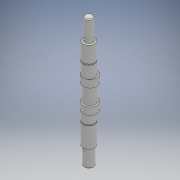
# Autodesk Inventor part: 도면2-4번
Saved by Autodesk Inventor 2018.3 (Build 223284000, 284)
## iProperties
Created: 2019-10-11
Part Number: 도면2-4번
Material: 일반
Document SubType Name: Modeling
Designer: MyTool
Density: 1 g/cm^3
Appearance: 기본값
Author: MyTool
Autodesk Inventor part; units mm, degrees
ref_plane "YZ Plane" through (0, 0, 0) normal (1, 0, 0) x (0, 1, 0)
ref_plane "XZ Plane" through (0, 0, 0) normal (0, 1, 0) x (-1, 0, 0)
ref_plane "XY Plane" through (0, 0, 0) normal (0, 0, 1) x (1, 0, 0)
sketch "스케치1" plane through (0, 0, 0) normal (1, 0, 0) x (0, 1, 0)
  line L0 (0, 0) -> (6, 0)
  line L1 (6, 0) -> (6, 23)
  line L2 (6, 23) -> (0, 23)
  line L3 (0, 23) -> (0, 0)
  line L4 (0, 23) -> (7.5, 23)
  line L5 (7.5, 23) -> (7.5, 61)
  line L6 (7.5, 61) -> (0, 61)
  line L7 (0, 61) -> (0, 23)
  line L8 (0, 61) -> (10.5, 61)
  line L9 (10.5, 61) -> (10.5, 70.5)
  line L10 (10.5, 70.5) -> (0, 70.5)
  line L11 (0, 70.5) -> (0, 61)
  line L12 (0, 70.5) -> (12.5, 70.5)
  line L13 (12.5, 70.5) -> (12.5, 91.5)
  line L14 (12.5, 91.5) -> (0, 91.5)
  line L15 (0, 91.5) -> (0, 70.5)
  line L16 (0, 91.5) -> (10.5, 91.5)
  line L17 (10.5, 91.5) -> (10.5, 101)
  line L18 (10.5, 101) -> (0, 101)
  line L19 (0, 101) -> (0, 91.5)
  line L20 (0, 101) -> (7.5, 101)
  line L21 (7.5, 101) -> (7.5, 139)
  line L22 (7.5, 139) -> (0, 139)
  line L23 (0, 139) -> (0, 101)
  line L24 (0, 139) -> (5, 139)
  line L25 (5, 139) -> (5, 166)
  line L26 (5, 166) -> (0, 166)
  line L27 (0, 166) -> (0, 139)
  dimension "d0" = 23
  dimension "d1" = 38
  dimension "d2" = 9.5
  dimension "d3" = 21
  dimension "d4" = 9.5
  dimension "d5" = 38
  dimension "d6" = 27
  dimension "d7" = 12
  dimension "d8" = 15
  dimension "d9" = 21
  dimension "d10" = 25
  dimension "d11" = 10
  constraints: 56 end point, 14 parallel, 7 horizontal, 7 perpendicular, 2 point on line
  measures "d0" distance of L0.end L1.end
  measures "d1" distance of L4.end L5.end
  measures "d2" distance of L8.end L9.end
  measures "d3" distance of L12.end L13.end
  measures "d4" distance of L16.end L17.end
  measures "d5" distance of L20.end L21.end
  measures "d6" distance of L24.end L25.end
  measures "d7" diameter of L1 L3
  measures "d8" diameter of L5 L7
  measures "d9" diameter of L9 L11
  measures "d10" diameter of L13 L15
  measures "d11" diameter of L25 L27
revolve "회전1" add sketch "스케치1" angle 360 about axis through (0, 0, 23) along (0, 0, -1)
sketch "스케치3" plane through (0, 0, 101) normal (0, 0, 1) x (1, 0, 0)
  circle A0 centre (0, 0) radius 7.5 projected
  circle A1 centre (0, 1.5) radius 9
  circle A2 centre (0, 0) radius 10.5 projected
  dimension "d13" = 18
  constraints: 1 centre point, 1 tangent
  measures "d13" diameter of A1
extrude "돌출1" cut sketch "스케치3" against normal blind 9.5 contours A2
sketch "스케치2" plane through (0, 0, 61) normal (0, 0, -1) x (-1, 0, 0)
  circle A0 centre (0, 1.5) radius 9 projected
  circle A1 centre (0, 0) radius 10.5 projected
  point P0 (0, -7.5)
  constraints: 1 vertical alignment
extrude "돌출2" cut sketch "스케치2" against normal blind 9.5
sketch "스케치4" plane through (0, 0, 70.5) normal (0, 0, -1) x (-1, 0, 0)
  circle A0 centre (0, 1.5) radius 9 projected
  circle A1 centre (0, 1.5) radius 7
  circle A2 centre (0, 0) radius 12.5 projected
  point P0 (0, -7.5)
  dimension "d18" = 14
  constraints: 1 centre point, 1 coincident, 1 vertical alignment
  measures "d18" diameter of A1
extrude "돌출3" cut sketch "스케치4" against normal blind 21 contours A0 | A2
sketch "스케치5" plane through (0, 0, 0) normal (1, 0, 0) x (0, 1, 0)
  line L0 (7.5, 61) -> (7.5, 23) projected
  line L1 (7.5, 49) -> (7, 49)
  line L2 (7, 49) -> (7, 50.35)
  line L3 (7, 50.35) -> (7.5, 50.35)
  line L4 (7.5, 50.35) -> (7.5, 49)
  line L5 (7.5, 139) -> (7.5, 101) projected
  line L6 (7.5, 116.65) -> (7, 116.65)
  line L7 (7, 116.65) -> (7, 118)
  line L8 (7, 118) -> (7.5, 118)
  line L9 (7.5, 118) -> (7.5, 116.65)
  line L10 (0, -27.8) -> (0, 166.8) projected
  point P0 (0, 0)
  dimension "d22" = 0.5
  dimension "d23" = 1.35
  dimension "d24" = 0.5
  dimension "d25" = 26
  dimension "d26" = 0.5
  dimension "d27" = 1.35
  dimension "d28" = 21
  constraints: 16 end point, 3 perpendicular, 3 point on line, 2 horizontal, 2 parallel
  measures "d22" distance of L1.start L1.end
  measures "d23" distance of L1.end L2.end
  measures "d24" distance of L2.end L3.end
  measures "d25" distance from line of L0.end L1
  measures "d26" distance of L7.end L8.end
  measures "d27" distance of L6.end L7.end
  measures "d28" distance of L5.start L8.end
revolve "회전2" cut sketch "스케치5" angle 360 about axis through (0, 0, -10) along (0, 0, 1)
sketch "스케치6" plane through (0, 0, 0) normal (1, 0, 0) x (0, 1, 0)
  line L0 (-6, 23) -> (-6, 0) projected
  line L1 (-6, 20) -> (-6, 18.5)
  line L2 (-6, 18.5) -> (-4.5, 20)
  line L3 (-4.5, 20) -> (-6, 20)
  point P0 (0, 0)
  dimension "d31" = 1.5
  dimension "d32" = 1.5
  dimension "d33" = 3
  constraints: 6 end point, 2 point on line, 1 perpendicular
  measures "d31" distance of L1.start L1.end
  measures "d32" distance of L2.end L1.start
  measures "d33" distance from line of L0.start L3
revolve "회전3" cut sketch "스케치6" angle 360 about axis through (0, -4.5, 20) along (0, -1, 0)
sketch "스케치7" plane through (0, 0, 0) normal (1, 0, 0) x (0, 1, 0)
  line L0 (-5, 141.5) -> (-5, 143)
  line L1 (-5, 143) -> (-3.5, 143)
  line L2 (-3.5, 143) -> (-5, 141.5)
  line L3 (-5, 166) -> (-5, 139) projected
  point P0 (0, 0)
  dimension "d37" = 1.5
  dimension "d38" = 1.5
  dimension "d39" = 4
  constraints: 6 end point, 1 collinear, 1 perpendicular, 1 vertical
  measures "d37" distance of L0.start L0.end
  measures "d38" distance of L0.end L1.end
  measures "d39" distance of L0.end L3.end
revolve "회전4" cut sketch "스케치7" angle 360 about axis through (0, -5, 143) along (0, 1, 0)
sketch "스케치8" plane through (0, 0, 0) normal (1, 0, 0) x (0, 1, 0)
  circle A0 centre (8.7, 13) radius 8
  line L0 (6, 23) -> (6, 0) projected
  circle A1 centre (7.7, 151) radius 6.5
  line L1 (5, 166) -> (5, 139) projected
  line L2 (-5, 139) -> (5, 139) projected
  point P0 (0, 0)
  dimension "d41" = 16
  dimension "d42" = 5.3
  dimension "d43" = 10
  dimension "d44" = 13
  dimension "d45" = 3.8
  dimension "d47" = 12
  constraints: 2 centre point
  measures "d41" diameter of A0
  measures "d42" distance edge to line of A0 L0
  measures "d43" vertical distance of L0.start A0.centre
  measures "d44" diameter of A1
  measures "d45" distance edge to line of A1 L1
  measures "d47" distance from line of A1.centre L2
extrude "돌출4" cut sketch "스케치8" along normal mid plane 3
chamfer "모따기1" distance 1 angle 45 2 edges at (0, -6, 0) (0, -5, 166)
equation "\"d4\" = d2"
equation "\"d5\" = d1"
